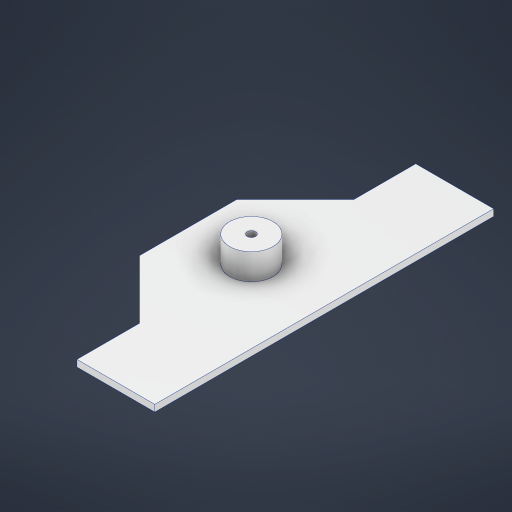
# Autodesk Inventor part: XAxisCreplCaretki
Saved by Autodesk Inventor 2024 (Build 280153000, 153)
## iProperties
Created: 2023-12-22
Part Number: XAxisCreplCaretki
Material: Aluminum 6061
Document SubType Name: Modeling
Designer: KirikDK
Mass: 2500.41 g
Surface Area: 1830.34 cm^2
Volume: 926.078 cm^3
Density: 2.7 g/cm^3
Appearance: Aluminum - Flat
Author: KirikDK
Autodesk Inventor part; units mm, degrees
ref_plane "YZ Plane" through (0, 0, 0) normal (1, 0, 0) x (0, 1, 0)
ref_plane "XZ Plane" through (0, 0, 0) normal (0, 1, 0) x (-1, 0, 0)
ref_plane "XY Plane" through (0, 0, 0) normal (0, 0, 1) x (1, 0, 0)
sketch "Sketch1" plane through (0, 0, 0) normal (0, 1, 0) x (-1, 0, 0)
  line L0 (-102.1567, -250.3174) -> (-102.1567, 267.6805)
  line L1 (-102.1567, -246.3184) -> (-102.1567, 262.6816)
  line L2 (-102.1567, 262.6816) -> (14.8433, 262.6816)
  line L3 (102.8433, 80.6816) -> (14.8433, 168.6816)
  line L4 (14.8433, 262.6816) -> (14.8433, 168.6816)
  line L5 (14.8433, 168.6816) -> (102.8433, 80.6816)
  line L6 (102.8433, 80.6816) -> (102.8433, -65.3184)
  line L7 (102.8433, -65.3184) -> (14.8433, -153.3184)
  line L8 (14.8433, -153.3184) -> (14.8433, -246.3184)
  line L9 (14.8433, -246.3184) -> (-102.1567, -246.3184)
  point P0 (0, 0)
  point P1 (-37.1567, -11.3184)
  dimension "d0" = 509
  dimension "d1" = 117
  dimension "d2" = 117
  dimension "d3" = 93
  dimension "d4" = 94
  dimension "d6" = 88
  dimension "d7" = 88
  dimension "d8" = 88
  dimension "d9" = 88
  constraints: 20 end point, 4 point on line, 2 perpendicular, 1 collinear, 1 parallel, 1 vertical
  measures "d0" distance of L1.start L1.end
  measures "d1" distance of L1.end L4.start
  measures "d2" distance of L8.end L1.start
  measures "d3" distance of L8.start L8.end
  measures "d4" distance of L4.start L3.end
  measures "d6" horizontal distance of L6.start L3.end
  measures "d7" horizontal distance of L6.start L3.end
  measures "d8" horizontal distance of L7.start L8.start
  measures "d9" horizontal distance of L7.start L8.start
extrude "Extrusion1" add sketch "Sketch1" along normal blind 10
sketch "Sketch2" plane through (0, 10, 0) normal (0, 1, 0) x (1, 0, 0)
  line L0 (-102.8433, 65.3184) -> (-102.8433, -80.6816) projected
  circle A0 centre (-102.8433, -7.6816) radius 9.3184
  circle A1 centre (-7.8433, -7.6816) radius 32.5
  circle A2 centre (-7.8433, -7.6816) radius 6.25
  line L1 (102.1567, -262.6816) -> (102.1567, 246.3184) projected
  line L2 (102.1567, 246.3184) -> (-14.8433, 246.3184) projected
  point P0 (0, 0)
  dimension "d14" = 95
  dimension "d16" = 254
  dimension "d17" = 110
  dimension "d18" = 65
  dimension "d19" = 12.5
  constraints: 3 centre point, 2 midpoint, 1 coincident
  measures "d14" distance of point (-102.843, -7.682) A1.centre
  measures "d16" distance from line of L2 A1.centre
  measures "d17" distance from line of L1 A1.centre
  measures "d18" diameter of A1
  measures "d19" diameter of A2
extrude "Extrusion2" add sketch "Sketch2" along normal blind 39 contours A1
body "Solid1"
